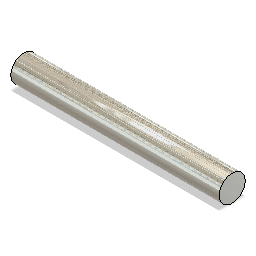
GuardaLamas_1 (Autodesk Fusion 360 archive; units mm, degrees)
design "Shaft2"
Autodesk Fusion 360 part; units mm, degrees
sketch "Sketch1" plane through (0, 0, 0) normal (1, 0, 0) x (0, 0, -1)
  circle A0 centre (0, 0) radius 1.5
  dimension "d1" = 3
  constraint coincident A0.centre origin
  measures "d1" diameter of A0
extrude "Extrude1" add sketch "Sketch1" along normal blind 23.5
extrude "Extrude2" add 1 faces at (0, -0.5383, -0.567) along direction (-1, 0, 0) blind 0.5

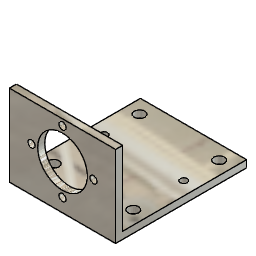
design "chapinhas"
Autodesk Fusion 360 part; units mm, degrees
sketch "Sketch1" plane through (0, 0, 0) normal (0, 0, 1) x (1, 0, 0)
  circle A0 centre (0, 0) radius 14
  circle A1 centre (17.5, 0) radius 2
  circle A2 centre (0, 17.5) radius 2
  circle A3 centre (-17.5, 0) radius 2
  circle A4 centre (0, -17.5) radius 2
  line L0 (30, -21) -> (-30, -21)
  line L1 (-30, -21) -> (-30, 21)
  line L2 (-30, 21) -> (30, 21)
  line L3 (30, 21) -> (30, -21)
  line L4 (-30, -21) -> (30, -21)
  line L5 (30, -21) -> (30, -25)
  line L6 (30, -25) -> (-30, -25)
  line L7 (-30, -25) -> (-30, -21)
  dimension "d2" = 28
  dimension "d4" = 4
  dimension "d6" = 360
  dimension "d7" = 60
  dimension "d8" = 42
  dimension "d9" = 60
  dimension "d10" = 4
  constraint horizontal L0
  constraint perpendicular L0 L1
  constraint parallel L0 L2
  constraint parallel L1 L3
  constraint coincident A0.centre origin
  constraint horizontal L4
  constraint vertical L5
  constraint horizontal L6
  constraint vertical L7
  measures "d2" diameter of A0
  measures "d4" diameter of A1
  measures "d4" distance of L0.end L6.end
extrude "Extrude1" add sketch "Sketch1" along normal blind 4
extrude "Extrude2" add sketch "Sketch1" against normal blind 70 contours L0 L4 L5 L6 L7
sketch "Sketch2" plane through (0, -25, 0) normal (0, -1, 0) x (1, 0, 0)
  line L0 (30, -70) -> (30, 4)
  line L1 (30, 4) -> (-30, 4)
  line L2 (-30, 4) -> (-30, -70)
  line L3 (-30, -70) -> (30, -70)
  circle A0 centre (-22.5, -13.5) radius 3
  circle A1 centre (-22.5, -42) radius 2
  circle A2 centre (-22.5, -62) radius 3
  circle A3 centre (22.5, -42) radius 2
  circle A4 centre (22.5, -62) radius 3
  circle A5 centre (22.5, -13.5) radius 3
  dimension "d24" = 6
  dimension "d25" = 4
  dimension "d26" = 6
  measures "d24" diameter of A0
  measures "d4" diameter of A1
  measures "d26" diameter of A2
extrude "Extrude3" cut sketch "Sketch2" against normal blind 10 contours A0 | A1 | A2 | A3 | A4 | A5
equation "d11 = d10"

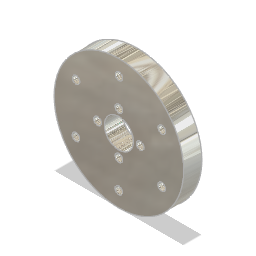
design "Espacador"
Autodesk Fusion 360 part; units mm, degrees
sketch "Sketch1" plane through (0, 0, 0) normal (0, 0, 1) x (-1, 0, 0)
  circle A0 centre (0, 0) radius 9.55
  circle A1 centre (0, 0) radius 32.5
  circle A2 centre (-0.0863, -32.4999) radius 2.5
  circle A3 centre (28.1026, -16.3247) radius 2.5
  circle A4 centre (28.1889, 16.1752) radius 2.5
  circle A5 centre (0.0863, 32.4999) radius 2.5
  circle A6 centre (-28.1026, 16.3247) radius 2.5
  circle A7 centre (-28.1889, -16.1752) radius 2.5
  circle A8 centre (0, 0) radius 42.5
  dimension "d1" = 19.1
  dimension "d4" = 65
  dimension "d5" = 5
  dimension "d7" = 360
  dimension "d9" = 85
  constraint concentric A0 A1
  constraint coincident A1 A2.centre
  constraint concentric A1 A8
  measures "d1" diameter of A0
  measures "d4" diameter of A1
  measures "d5" diameter of A2
  measures "d9" diameter of A8
extrude "Extrude1" add sketch "Sketch1" along normal blind 12 contours A1 A2 A3 A4 A5 A6 A7 | A8
sketch "Sketch2" plane through (0, 0, 12) normal (0, 0, 1) x (1, 0, 0)
  circle A0 centre (28.1026, -16.3247) radius 2.5
  circle A1 centre (0.0863, 32.4999) radius 2.5
  circle A2 centre (-0.0863, -32.4999) radius 2.5
  circle A3 centre (28.1889, 16.1752) radius 2.5
  circle A4 centre (-28.1026, 16.3247) radius 2.5
  circle A5 centre (-28.1889, -16.1752) radius 2.5
  circle A6 centre (0, 0) radius 9.55
  circle A7 centre (0, 0) radius 42.5
  circle A8 centre (0, 0) radius 14
  circle A9 centre (14, 0) radius 2.55
  circle A10 centre (0, 14) radius 2.55
  circle A11 centre (-14, 0) radius 2.55
  circle A12 centre (0, -14) radius 2.55
  dimension "d10" = 28
  dimension "d11" = 5.1
  dimension "d13" = 360
  constraint coincident A6.centre A7.centre
  constraint coincident A8 A9.centre
  measures "d10" diameter of A8
  measures "d11" diameter of A9
extrude "Extrude2" cut sketch "Sketch2" against normal blind 31 contours A8 A9 | A8 A9 | A8 A10 | A8 A10 | A8 A12 | A8 A12 | A8 A11 | A8 A11

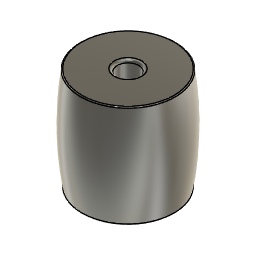
design "Borracha_roda"
Autodesk Fusion 360 part; units mm, degrees
sketch "Esboço1" plane through (0, 0, 0) normal (1, 0, 0) x (0, 1, 0)
  line L0 (0, 0) -> (8.5, 0)
  line L1 (0, 0) -> (0, 19)
  line L2 (0, 19) -> (8.7, 19)
  arc A0 (8.5, 0) -> (8.7, 19) centre (-53.1703, 10.1502) ccw
  line L3 (8.5, 0) -> (8.5, 10.6447)
  dimension "d1" = 8.5
  dimension "d2" = 19
  dimension "d3" = 8.7
  dimension "d5" = 125
  constraint coincident L0.start L1.start
  constraint horizontal L0
  constraint perpendicular L0 L1
  constraint perpendicular L1 L2
  constraint perpendicular L0 L3
  measures "d1" distance of L0.start L0.end
  measures "d2" distance of L0.start L1.end
  measures "d3" distance of L1.end L2.end
  measures "d5" diameter of A0
revolve "Revolucionar1" add sketch "Esboço1" angle 360 about axis through (0, 0, 0) along (0, 0, 1)
sketch "Esboço2" plane through (0, 0, 19) normal (0, 0, 1) x (-1, 0, 0)
  circle A0 centre (0, 0) radius 8.7
  circle A1 centre (0, 0) radius 2
  dimension "d7" = 4
  constraint concentric A0 A1
  measures "d7" diameter of A1
extrude "Extrusão1" cut sketch "Esboço2" against normal blind 24 contours A1
fillet "Arredondamento1" radius 0.5 2 edges at (1.8647, -0.7232, 19) (1.8647, 0.7232, 0)
fillet "Arredondamento2" radius 0.2 2 edges at (-8.1112, 3.1461, 19) (-7.9248, 3.0737, 0)

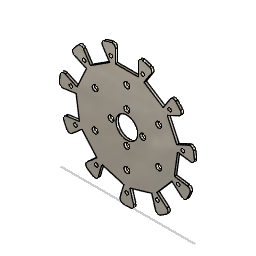
design "Disc Baixo" references "Shaft2"
Autodesk Fusion 360 part; units mm, degrees
sketch "Sketch3" plane through (0, 0, 0) normal (0, 0, 1) x (-1, 0, 0)
  arc A0 (-58.8397, -11.7426) -> (-54.6515, -13.8844) centre (-55.8977, -11.1555) ccw
  line L0 (-54.6515, -13.8844) -> (-44.1121, -9.0712)
  line L1 (-44.1121, -9.0712) -> (-35.7428, -27.3974)
  line L2 (-35.7428, -27.3974) -> (-46.2822, -32.2105)
  arc A1 (-46.2822, -32.2105) -> (-47.4063, -36.7783) centre (-45.036, -34.9394) ccw
  arc A2 (-47.4063, -36.7783) -> (-43.1506, -41.6896) centre (0, 0) ccw
  arc A3 (-43.1506, -41.6896) -> (-38.4693, -41.2271) centre (-40.9931, -39.6052) ccw
  line L3 (-38.4693, -41.2271) -> (-32.2052, -31.48)
  line L4 (-32.2052, -31.48) -> (-15.2567, -42.3722)
  line L5 (-15.2567, -42.3722) -> (-21.5207, -52.1193)
  arc A4 (-21.5207, -52.1193) -> (-19.9968, -56.5697) centre (-18.997, -53.7412) ccw
  arc A5 (-19.9968, -56.5697) -> (-13.7615, -58.4005) centre (0, 0) ccw
  arc A6 (-13.7615, -58.4005) -> (-10.0734, -55.4805) centre (-13.0734, -55.4805) ccw
  line L6 (-10.0734, -55.4805) -> (-10.0734, -43.8941)
  line L7 (-10.0734, -43.8941) -> (10.0734, -43.8941)
  line L8 (10.0734, -43.8941) -> (10.0734, -55.4805)
  arc A7 (10.0734, -55.4805) -> (13.7615, -58.4005) centre (13.0734, -55.4805) ccw
  arc A8 (13.7615, -58.4005) -> (19.9968, -56.5697) centre (0, 0) ccw
  arc A9 (19.9968, -56.5697) -> (21.5207, -52.1193) centre (18.997, -53.7412) ccw
  line L9 (21.5207, -52.1193) -> (15.2567, -42.3722)
  line L10 (15.2567, -42.3722) -> (32.2052, -31.48)
  line L11 (32.2052, -31.48) -> (38.4693, -41.2271)
  arc A10 (38.4693, -41.2271) -> (43.1506, -41.6896) centre (40.9931, -39.6052) ccw
  arc A11 (43.1506, -41.6896) -> (47.4063, -36.7783) centre (0, 0) ccw
  arc A12 (47.4063, -36.7783) -> (46.2822, -32.2105) centre (45.036, -34.9394) ccw
  line L12 (46.2822, -32.2105) -> (35.7428, -27.3974)
  line L13 (35.7428, -27.3974) -> (44.1121, -9.0712)
  line L14 (44.1121, -9.0712) -> (54.6515, -13.8844)
  arc A13 (54.6515, -13.8844) -> (58.8397, -11.7426) centre (55.8977, -11.1555) ccw
  arc A14 (58.8397, -11.7426) -> (59.7646, -5.3101) centre (0, 0) ccw
  arc A15 (59.7646, -5.3101) -> (56.3494, -2.0752) centre (56.7763, -5.0446) ccw
  line L15 (56.3494, -2.0752) -> (44.8809, -3.7241)
  line L16 (44.8809, -3.7241) -> (42.0137, 16.2176)
  line L17 (42.0137, 16.2176) -> (53.4822, 17.8666)
  arc A16 (53.4822, 17.8666) -> (55.8476, 21.9327) centre (53.0553, 20.836) ccw
  arc A17 (55.8476, 21.9327) -> (53.148, 27.844) centre (0, 0) ccw
  arc A18 (53.148, 27.844) -> (48.526, 28.719) centre (50.4906, 26.4518) ccw
  line L18 (48.526, 28.719) -> (39.7696, 21.1316)
  line L19 (39.7696, 21.1316) -> (26.5763, 36.3575)
  line L20 (26.5763, 36.3575) -> (35.3327, 43.945)
  arc A19 (35.3327, 43.945) -> (35.1243, 48.6444) centre (33.3681, 46.2122) ccw
  arc A20 (35.1243, 48.6444) -> (29.6574, 52.1578) centre (0, 0) ccw
  arc A21 (29.6574, 52.1578) -> (25.296, 50.3952) centre (28.1745, 49.55) ccw
  line L21 (25.296, 50.3952) -> (22.0318, 39.2781)
  line L22 (22.0318, 39.2781) -> (2.701, 44.9541)
  line L23 (2.701, 44.9541) -> (5.9653, 56.0712)
  arc A22 (5.9653, 56.0712) -> (3.2493, 59.912) centre (3.0868, 56.9164) ccw
  arc A23 (3.2493, 59.912) -> (-3.2493, 59.912) centre (0, 0) ccw
  arc A24 (-3.2493, 59.912) -> (-5.9653, 56.0712) centre (-3.0868, 56.9164) ccw
  line L24 (-5.9653, 56.0712) -> (-2.701, 44.9541)
  line L25 (-2.701, 44.9541) -> (-22.0318, 39.2781)
  line L26 (-22.0318, 39.2781) -> (-25.296, 50.3952)
  arc A25 (-25.296, 50.3952) -> (-29.6574, 52.1578) centre (-28.1745, 49.55) ccw
  arc A26 (-29.6574, 52.1578) -> (-35.1243, 48.6444) centre (0, 0) ccw
  arc A27 (-35.1243, 48.6444) -> (-35.3327, 43.945) centre (-33.3681, 46.2122) ccw
  line L27 (-35.3327, 43.945) -> (-26.5763, 36.3575)
  line L28 (-26.5763, 36.3575) -> (-39.7696, 21.1316)
  line L29 (-39.7696, 21.1316) -> (-48.526, 28.719)
  arc A28 (-48.526, 28.719) -> (-53.148, 27.844) centre (-50.4906, 26.4518) ccw
  arc A29 (-53.148, 27.844) -> (-55.8476, 21.9327) centre (0, 0) ccw
  arc A30 (-55.8476, 21.9327) -> (-53.4822, 17.8666) centre (-53.0553, 20.836) ccw
  line L30 (-53.4822, 17.8666) -> (-42.0137, 16.2176)
  line L31 (-42.0137, 16.2176) -> (-44.8809, -3.7241)
  line L32 (-44.8809, -3.7241) -> (-56.3494, -2.0752)
  arc A31 (-56.3494, -2.0752) -> (-59.7646, -5.3101) centre (-56.7763, -5.0446) ccw
  arc A32 (-59.7646, -5.3101) -> (-58.8397, -11.7426) centre (0, 0) ccw
  circle A33 centre (-45.4816, 20.7708) radius 1.5
  circle A34 centre (-27.032, 42.0627) radius 1.5
  circle A35 centre (0, 50) radius 1.5
  circle A36 centre (27.032, 42.0627) radius 1.5
  circle A37 centre (45.4816, 20.7708) radius 1.5
  circle A38 centre (49.4911, -7.1157) radius 1.5
  circle A39 centre (37.7875, -32.743) radius 1.5
  circle A40 centre (14.0866, -47.9746) radius 1.5
  circle A41 centre (-49.4911, -7.1157) radius 1.5
  circle A42 centre (-37.7875, -32.743) radius 1.5
  circle A43 centre (-14.0866, -47.9746) radius 1.5
  circle A44 centre (12.5, -21.6506) radius 8
  circle A45 centre (-20.5681, -11.875) radius 2.6
  circle A46 centre (-20.5681, 11.875) radius 2.6
  circle A47 centre (0, 23.75) radius 2.6
  circle A48 centre (20.5681, 11.875) radius 2.6
  circle A49 centre (20.5681, -11.875) radius 2.6
  circle A50 centre (-12.5, -21.6506) radius 8
  circle A51 centre (0, -23.75) radius 2.6
  circle A52 centre (25, 0) radius 8
  circle A53 centre (12.5, 21.6506) radius 8
  circle A54 centre (-12.5, 21.6506) radius 8
  circle A55 centre (-25, 0) radius 8
  circle A56 centre (0, 0) radius 11
  circle A57 centre (0, 50) radius 1.5
extrude "Extrude2" add sketch "Sketch3" along normal blind 2 contours A0 L0 L1 L2 A1 A2 A3 L3 L4 L5 A4 A5 A6 L6 L7 L8 A7 A8 A9 L9 L10 L11 A10 A11 A12 L12 L13 L14 A13 A14 A15 L15 L16 L17 A16 A17 A18 L18 L19 L20 A19 A20 A21 L21 L22 L23 A22 A23 A24 L24 L25 L26 A25 A26 A27 L27 L28 L29 A28 A29 A30 L30 L31 L32 A31 A32 | A33 | A34 | A35 A57 | A36 | A37 | A38 | A39 | A40 | A41 | A42 | A43 | A44 | A45 | A46 | A47 | A48 | A49 | A50 | A51 | A52 | A53 | A54 | A55 | A56
component_pattern "component pattern"
move_body "Move2" bodies 1 to x (1, 0, 0) y (0, 1, 0) z (0, 0, 1) at (0, 0, -2)
combine "Combine3" [suppressed]
sketch "Sketch5" plane through (0, 0, -2) normal (0, 0, -1) x (-1, 0, 0)
  line L0 (54.6515, 13.8844) -> (44.1121, 9.0712)
  line L1 (44.1121, 9.0712) -> (35.7428, 27.3974)
  line L2 (35.7428, 27.3974) -> (46.2822, 32.2105)
  arc A0 (46.2822, 32.2105) -> (47.4063, 36.7783) centre (45.036, 34.9394) ccw
  arc A1 (47.4063, 36.7783) -> (43.1506, 41.6896) centre (0, 0) ccw
  arc A2 (43.1506, 41.6896) -> (38.4693, 41.2271) centre (40.9931, 39.6052) ccw
  line L3 (38.4693, 41.2271) -> (32.2052, 31.48)
  line L4 (32.2052, 31.48) -> (15.2567, 42.3722)
  line L5 (15.2567, 42.3722) -> (21.5207, 52.1193)
  arc A3 (21.5207, 52.1193) -> (19.9968, 56.5697) centre (18.997, 53.7412) ccw
  arc A4 (19.9968, 56.5697) -> (13.7615, 58.4005) centre (0, 0) ccw
  arc A5 (13.7615, 58.4005) -> (10.0734, 55.4805) centre (13.0734, 55.4805) ccw
  line L6 (10.0734, 55.4805) -> (10.0734, 43.8941)
  line L7 (10.0734, 43.8941) -> (-10.0734, 43.8941)
  line L8 (-10.0734, 43.8941) -> (-10.0734, 55.4805)
  arc A6 (-10.0734, 55.4805) -> (-13.7615, 58.4005) centre (-13.0734, 55.4805) ccw
  arc A7 (-13.7615, 58.4005) -> (-19.9968, 56.5697) centre (0, 0) ccw
  arc A8 (-19.9968, 56.5697) -> (-21.5207, 52.1193) centre (-18.997, 53.7412) ccw
  line L9 (-21.5207, 52.1193) -> (-15.2567, 42.3722)
  line L10 (-15.2567, 42.3722) -> (-32.2052, 31.48)
  line L11 (-32.2052, 31.48) -> (-38.4693, 41.2271)
  arc A9 (-38.4693, 41.2271) -> (-43.1506, 41.6896) centre (-40.9931, 39.6052) ccw
  arc A10 (-43.1506, 41.6896) -> (-47.4063, 36.7783) centre (0, 0) ccw
  arc A11 (-47.4063, 36.7783) -> (-46.2822, 32.2105) centre (-45.036, 34.9394) ccw
  line L12 (-46.2822, 32.2105) -> (-35.7428, 27.3974)
  line L13 (-35.7428, 27.3974) -> (-44.1121, 9.0712)
  line L14 (-44.1121, 9.0712) -> (-54.6515, 13.8844)
  arc A12 (-54.6515, 13.8844) -> (-58.8397, 11.7426) centre (-55.8977, 11.1555) ccw
  arc A13 (-58.8397, 11.7426) -> (-59.7646, 5.3101) centre (0, 0) ccw
  arc A14 (-59.7646, 5.3101) -> (-56.3494, 2.0752) centre (-56.7763, 5.0446) ccw
  line L15 (-56.3494, 2.0752) -> (-44.8809, 3.7241)
  line L16 (-44.8809, 3.7241) -> (-42.0137, -16.2176)
  line L17 (-42.0137, -16.2176) -> (-53.4822, -17.8666)
  arc A15 (-53.4822, -17.8666) -> (-55.8476, -21.9327) centre (-53.0553, -20.836) ccw
  arc A16 (-55.8476, -21.9327) -> (-53.148, -27.844) centre (0, 0) ccw
  arc A17 (-53.148, -27.844) -> (-48.526, -28.719) centre (-50.4906, -26.4518) ccw
  line L18 (-48.526, -28.719) -> (-39.7696, -21.1316)
  line L19 (-39.7696, -21.1316) -> (-26.5763, -36.3575)
  line L20 (-26.5763, -36.3575) -> (-35.3327, -43.945)
  arc A18 (-35.3327, -43.945) -> (-35.1243, -48.6444) centre (-33.3681, -46.2122) ccw
  arc A19 (-35.1243, -48.6444) -> (-29.6574, -52.1578) centre (0, 0) ccw
  arc A20 (-29.6574, -52.1578) -> (-25.296, -50.3952) centre (-28.1745, -49.55) ccw
  line L21 (-25.296, -50.3952) -> (-22.0318, -39.2781)
  line L22 (-22.0318, -39.2781) -> (-2.701, -44.9541)
  line L23 (-2.701, -44.9541) -> (-5.9653, -56.0712)
  arc A21 (-5.9653, -56.0712) -> (-3.2493, -59.912) centre (-3.0868, -56.9164) ccw
  arc A22 (-3.2493, -59.912) -> (3.2493, -59.912) centre (0, 0) ccw
  arc A23 (3.2493, -59.912) -> (5.9653, -56.0712) centre (3.0868, -56.9164) ccw
  line L24 (5.9653, -56.0712) -> (2.701, -44.9541)
  line L25 (2.701, -44.9541) -> (22.0318, -39.2781)
  line L26 (22.0318, -39.2781) -> (25.296, -50.3952)
  arc A24 (25.296, -50.3952) -> (29.6574, -52.1578) centre (28.1745, -49.55) ccw
  arc A25 (29.6574, -52.1578) -> (35.1243, -48.6444) centre (0, 0) ccw
  arc A26 (35.1243, -48.6444) -> (35.3327, -43.945) centre (33.3681, -46.2122) ccw
  line L27 (35.3327, -43.945) -> (26.5763, -36.3575)
  line L28 (26.5763, -36.3575) -> (39.7696, -21.1316)
  line L29 (39.7696, -21.1316) -> (48.526, -28.719)
  arc A27 (48.526, -28.719) -> (53.148, -27.844) centre (50.4906, -26.4518) ccw
  arc A28 (53.148, -27.844) -> (55.8476, -21.9327) centre (0, 0) ccw
  arc A29 (55.8476, -21.9327) -> (53.4822, -17.8666) centre (53.0553, -20.836) ccw
  line L30 (53.4822, -17.8666) -> (42.0137, -16.2176)
  line L31 (42.0137, -16.2176) -> (44.8809, 3.7241)
  line L32 (44.8809, 3.7241) -> (56.3494, 2.0752)
  arc A30 (56.3494, 2.0752) -> (59.7646, 5.3101) centre (56.7763, 5.0446) ccw
  arc A31 (59.7646, 5.3101) -> (58.8397, 11.7426) centre (0, 0) ccw
  arc A32 (58.8397, 11.7426) -> (54.6515, 13.8844) centre (55.8977, 11.1555) ccw
  circle A33 centre (0, 0) radius 9.6
  circle A34 centre (0, 0) radius 32.5
  circle A35 centre (0, -32.5) radius 2.55
  circle A36 centre (28.1458, -16.25) radius 2.55
  circle A37 centre (28.1458, 16.25) radius 2.55
  circle A38 centre (0, 32.5) radius 2.55
  circle A39 centre (-28.1458, 16.25) radius 2.55
  circle A40 centre (-28.1458, -16.25) radius 2.55
  dimension "d11" = 19.2
  dimension "d16" = 65
  dimension "d17" = 5.1
  dimension "d19" = 360
  constraint coincident A1.centre A4.centre
  constraint concentric A33 A34
  constraint coincident A34 A35.centre
  measures "d11" diameter of A33
  measures "d16" diameter of A34
  measures "d17" diameter of A35
extrude "Extrude4" cut sketch "Sketch5" against normal blind 10 contours A33 | A34 A37 | A34 A37 | A34 A36 | A34 A36 | A34 A38 | A34 A38 | A34 A35 | A34 A35 | A34 A39 | A34 A39 | A34 A40 | A34 A40
sketch "Sketch6" plane through (0, 0, -2) normal (0, 0, -1) x (-1, 0, 0)
  circle A0 centre (0, 32.5) radius 2.55
  circle A1 centre (0, 0) radius 9.6
  circle A2 centre (28.1458, 16.25) radius 2.55
  circle A3 centre (-28.1458, 16.25) radius 2.55
  circle A4 centre (0, -32.5) radius 2.55
  circle A5 centre (28.1458, -16.25) radius 2.55
  circle A6 centre (-28.1458, -16.25) radius 2.55
  arc A7 (-58.8397, 11.7426) -> (-59.7646, 5.3101) centre (0, 0) ccw
  arc A8 (-59.7646, 5.3101) -> (-56.3494, 2.0752) centre (-56.7763, 5.0446) ccw
  line L0 (-56.3494, 2.0752) -> (-44.8809, 3.7241)
  line L1 (-44.8809, 3.7241) -> (-42.0137, -16.2176)
  line L2 (-42.0137, -16.2176) -> (-53.4822, -17.8666)
  arc A9 (-53.4822, -17.8666) -> (-55.8476, -21.9327) centre (-53.0553, -20.836) ccw
  arc A10 (-55.8476, -21.9327) -> (-53.148, -27.844) centre (0, 0) ccw
  arc A11 (-53.148, -27.844) -> (-48.526, -28.719) centre (-50.4906, -26.4518) ccw
  line L3 (-48.526, -28.719) -> (-39.7696, -21.1316)
  line L4 (-39.7696, -21.1316) -> (-26.5763, -36.3575)
  line L5 (-26.5763, -36.3575) -> (-35.3327, -43.945)
  arc A12 (-35.3327, -43.945) -> (-35.1243, -48.6444) centre (-33.3681, -46.2122) ccw
  arc A13 (-35.1243, -48.6444) -> (-29.6574, -52.1578) centre (0, 0) ccw
  arc A14 (-29.6574, -52.1578) -> (-25.296, -50.3952) centre (-28.1745, -49.55) ccw
  line L6 (-25.296, -50.3952) -> (-22.0318, -39.2781)
  line L7 (-22.0318, -39.2781) -> (-2.701, -44.9541)
  line L8 (-2.701, -44.9541) -> (-5.9653, -56.0712)
  arc A15 (-5.9653, -56.0712) -> (-3.2493, -59.912) centre (-3.0868, -56.9164) ccw
  arc A16 (-3.2493, -59.912) -> (3.2493, -59.912) centre (0, 0) ccw
  arc A17 (3.2493, -59.912) -> (5.9653, -56.0712) centre (3.0868, -56.9164) ccw
  line L9 (5.9653, -56.0712) -> (2.701, -44.9541)
  line L10 (2.701, -44.9541) -> (22.0318, -39.2781)
  line L11 (22.0318, -39.2781) -> (25.296, -50.3952)
  arc A18 (25.296, -50.3952) -> (29.6574, -52.1578) centre (28.1745, -49.55) ccw
  arc A19 (29.6574, -52.1578) -> (35.1243, -48.6444) centre (0, 0) ccw
  arc A20 (35.1243, -48.6444) -> (35.3327, -43.945) centre (33.3681, -46.2122) ccw
  line L12 (35.3327, -43.945) -> (26.5763, -36.3575)
  line L13 (26.5763, -36.3575) -> (39.7696, -21.1316)
  line L14 (39.7696, -21.1316) -> (48.526, -28.719)
  arc A21 (48.526, -28.719) -> (53.148, -27.844) centre (50.4906, -26.4518) ccw
  arc A22 (53.148, -27.844) -> (55.8476, -21.9327) centre (0, 0) ccw
  arc A23 (55.8476, -21.9327) -> (53.4822, -17.8666) centre (53.0553, -20.836) ccw
  line L15 (53.4822, -17.8666) -> (42.0137, -16.2176)
  line L16 (42.0137, -16.2176) -> (44.8809, 3.7241)
  line L17 (44.8809, 3.7241) -> (56.3494, 2.0752)
  arc A24 (56.3494, 2.0752) -> (59.7646, 5.3101) centre (56.7763, 5.0446) ccw
  arc A25 (59.7646, 5.3101) -> (58.8397, 11.7426) centre (0, 0) ccw
  arc A26 (58.8397, 11.7426) -> (54.6515, 13.8844) centre (55.8977, 11.1555) ccw
  line L18 (54.6515, 13.8844) -> (44.1121, 9.0712)
  line L19 (44.1121, 9.0712) -> (35.7428, 27.3974)
  line L20 (35.7428, 27.3974) -> (46.2822, 32.2105)
  arc A27 (46.2822, 32.2105) -> (47.4063, 36.7783) centre (45.036, 34.9394) ccw
  arc A28 (47.4063, 36.7783) -> (43.1506, 41.6896) centre (0, 0) ccw
  arc A29 (43.1506, 41.6896) -> (38.4693, 41.2271) centre (40.9931, 39.6052) ccw
  line L21 (38.4693, 41.2271) -> (32.2052, 31.48)
  line L22 (32.2052, 31.48) -> (15.2567, 42.3722)
  line L23 (15.2567, 42.3722) -> (21.5207, 52.1193)
  arc A30 (21.5207, 52.1193) -> (19.9968, 56.5697) centre (18.997, 53.7412) ccw
  arc A31 (19.9968, 56.5697) -> (13.7615, 58.4005) centre (0, 0) ccw
  arc A32 (13.7615, 58.4005) -> (10.0734, 55.4805) centre (13.0734, 55.4805) ccw
  line L24 (10.0734, 55.4805) -> (10.0734, 43.8941)
  line L25 (10.0734, 43.8941) -> (-10.0734, 43.8941)
  line L26 (-10.0734, 43.8941) -> (-10.0734, 55.4805)
  arc A33 (-10.0734, 55.4805) -> (-13.7615, 58.4005) centre (-13.0734, 55.4805) ccw
  arc A34 (-13.7615, 58.4005) -> (-19.9968, 56.5697) centre (0, 0) ccw
  arc A35 (-19.9968, 56.5697) -> (-21.5207, 52.1193) centre (-18.997, 53.7412) ccw
  line L27 (-21.5207, 52.1193) -> (-15.2567, 42.3722)
  line L28 (-15.2567, 42.3722) -> (-32.2052, 31.48)
  line L29 (-32.2052, 31.48) -> (-38.4693, 41.2271)
  arc A36 (-38.4693, 41.2271) -> (-43.1506, 41.6896) centre (-40.9931, 39.6052) ccw
  arc A37 (-43.1506, 41.6896) -> (-47.4063, 36.7783) centre (0, 0) ccw
  arc A38 (-47.4063, 36.7783) -> (-46.2822, 32.2105) centre (-45.036, 34.9394) ccw
  line L30 (-46.2822, 32.2105) -> (-35.7428, 27.3974)
  line L31 (-35.7428, 27.3974) -> (-44.1121, 9.0712)
  line L32 (-44.1121, 9.0712) -> (-54.6515, 13.8844)
  arc A39 (-54.6515, 13.8844) -> (-58.8397, 11.7426) centre (-55.8977, 11.1555) ccw
  circle A40 centre (0, -50) radius 1.55
  circle A41 centre (27.032, -42.0627) radius 1.55
  circle A42 centre (45.4816, -20.7708) radius 1.55
  circle A43 centre (49.4911, 7.1157) radius 1.55
  circle A44 centre (37.7875, 32.743) radius 1.55
  circle A45 centre (14.0866, 47.9746) radius 1.55
  circle A46 centre (-14.0866, 47.9746) radius 1.55
  circle A47 centre (-37.7875, 32.743) radius 1.55
  circle A48 centre (-49.4911, 7.1157) radius 1.55
  circle A49 centre (-45.4816, -20.7708) radius 1.55
  circle A50 centre (-27.032, -42.0627) radius 1.55
  dimension "d20" = 3.1
  dimension "d22" = 360
  measures "d20" diameter of A40
extrude "Extrude6" cut sketch "Sketch6" against normal blind 20 contours A40 | A41 | A42 | A43 | A44 | A45 | A46 | A47 | A48 | A49 | A50
sketch "Sketch8" plane through (0, 0, 0) normal (0, 0, 1) x (1, 0, 0)
  circle A0 centre (49.4911, 7.1157) radius 1.55
  circle A1 centre (-37.7875, 32.743) radius 1.55
  circle A2 centre (0, -50) radius 1.55
  circle A3 centre (-49.4911, 7.1157) radius 1.55
  circle A4 centre (37.7875, 32.743) radius 1.55
  circle A5 centre (45.4816, -20.7708) radius 1.55
  circle A6 centre (-14.0866, 47.9746) radius 1.55
  circle A7 centre (-27.032, -42.0627) radius 1.55
  circle A8 centre (-45.4816, -20.7708) radius 1.55
  circle A9 centre (14.0866, 47.9746) radius 1.55
  circle A10 centre (27.032, -42.0627) radius 1.55
  circle A11 centre (0, 32.5) radius 2.55
  circle A12 centre (0, 0) radius 9.6
  circle A13 centre (-28.1458, 16.25) radius 2.55
  circle A14 centre (28.1458, 16.25) radius 2.55
  circle A15 centre (0, -32.5) radius 2.55
  circle A16 centre (-28.1458, -16.25) radius 2.55
  circle A17 centre (28.1458, -16.25) radius 2.55
  arc A18 (59.7646, 5.3101) -> (58.8397, 11.7426) centre (0, 0) ccw
  arc A19 (58.8397, 11.7426) -> (54.6515, 13.8844) centre (55.8977, 11.1555) ccw
  line L0 (54.6515, 13.8844) -> (44.1121, 9.0712)
  line L1 (44.1121, 9.0712) -> (35.7428, 27.3974)
  line L2 (35.7428, 27.3974) -> (46.2822, 32.2105)
  arc A20 (46.2822, 32.2105) -> (47.4063, 36.7783) centre (45.036, 34.9394) ccw
  arc A21 (47.4063, 36.7783) -> (43.1506, 41.6896) centre (0, 0) ccw
  arc A22 (43.1506, 41.6896) -> (38.4693, 41.2271) centre (40.9931, 39.6052) ccw
  line L3 (38.4693, 41.2271) -> (32.2052, 31.48)
  line L4 (32.2052, 31.48) -> (15.2567, 42.3722)
  line L5 (15.2567, 42.3722) -> (21.5207, 52.1193)
  arc A23 (21.5207, 52.1193) -> (19.9968, 56.5697) centre (18.997, 53.7412) ccw
  arc A24 (19.9968, 56.5697) -> (13.7615, 58.4005) centre (0, 0) ccw
  arc A25 (13.7615, 58.4005) -> (10.0734, 55.4805) centre (13.0734, 55.4805) ccw
  line L6 (10.0734, 55.4805) -> (10.0734, 43.8941)
  line L7 (10.0734, 43.8941) -> (-10.0734, 43.8941)
  line L8 (-10.0734, 43.8941) -> (-10.0734, 55.4805)
  arc A26 (-10.0734, 55.4805) -> (-13.7615, 58.4005) centre (-13.0734, 55.4805) ccw
  arc A27 (-13.7615, 58.4005) -> (-19.9968, 56.5697) centre (0, 0) ccw
  arc A28 (-19.9968, 56.5697) -> (-21.5207, 52.1193) centre (-18.997, 53.7412) ccw
  line L9 (-21.5207, 52.1193) -> (-15.2567, 42.3722)
  line L10 (-15.2567, 42.3722) -> (-32.2052, 31.48)
  line L11 (-32.2052, 31.48) -> (-38.4693, 41.2271)
  arc A29 (-38.4693, 41.2271) -> (-43.1506, 41.6896) centre (-40.9931, 39.6052) ccw
  arc A30 (-43.1506, 41.6896) -> (-47.4063, 36.7783) centre (0, 0) ccw
  arc A31 (-47.4063, 36.7783) -> (-46.2822, 32.2105) centre (-45.036, 34.9394) ccw
  line L12 (-46.2822, 32.2105) -> (-35.7428, 27.3974)
  line L13 (-35.7428, 27.3974) -> (-44.1121, 9.0712)
  line L14 (-44.1121, 9.0712) -> (-54.6515, 13.8844)
  arc A32 (-54.6515, 13.8844) -> (-58.8397, 11.7426) centre (-55.8977, 11.1555) ccw
  arc A33 (-58.8397, 11.7426) -> (-59.7646, 5.3101) centre (0, 0) ccw
  arc A34 (-59.7646, 5.3101) -> (-56.3494, 2.0752) centre (-56.7763, 5.0446) ccw
  line L15 (-56.3494, 2.0752) -> (-44.8809, 3.7241)
  line L16 (-44.8809, 3.7241) -> (-42.0137, -16.2176)
  line L17 (-42.0137, -16.2176) -> (-53.4822, -17.8666)
  arc A35 (-53.4822, -17.8666) -> (-55.8476, -21.9327) centre (-53.0553, -20.836) ccw
  arc A36 (-55.8476, -21.9327) -> (-53.148, -27.844) centre (0, 0) ccw
  arc A37 (-53.148, -27.844) -> (-48.526, -28.719) centre (-50.4906, -26.4518) ccw
  line L18 (-48.526, -28.719) -> (-39.7696, -21.1316)
  line L19 (-39.7696, -21.1316) -> (-26.5763, -36.3575)
  line L20 (-26.5763, -36.3575) -> (-35.3327, -43.945)
  arc A38 (-35.3327, -43.945) -> (-35.1243, -48.6444) centre (-33.3681, -46.2122) ccw
  arc A39 (-35.1243, -48.6444) -> (-29.6574, -52.1578) centre (0, 0) ccw
  arc A40 (-29.6574, -52.1578) -> (-25.296, -50.3952) centre (-28.1745, -49.55) ccw
  line L21 (-25.296, -50.3952) -> (-22.0318, -39.2781)
  line L22 (-22.0318, -39.2781) -> (-2.701, -44.9541)
  line L23 (-2.701, -44.9541) -> (-5.9653, -56.0712)
  arc A41 (-5.9653, -56.0712) -> (-3.2493, -59.912) centre (-3.0868, -56.9164) ccw
  arc A42 (-3.2493, -59.912) -> (3.2493, -59.912) centre (0, 0) ccw
  arc A43 (3.2493, -59.912) -> (5.9653, -56.0712) centre (3.0868, -56.9164) ccw
  line L24 (5.9653, -56.0712) -> (2.701, -44.9541)
  line L25 (2.701, -44.9541) -> (22.0318, -39.2781)
  line L26 (22.0318, -39.2781) -> (25.296, -50.3952)
  arc A44 (25.296, -50.3952) -> (29.6574, -52.1578) centre (28.1745, -49.55) ccw
  arc A45 (29.6574, -52.1578) -> (35.1243, -48.6444) centre (0, 0) ccw
  arc A46 (35.1243, -48.6444) -> (35.3327, -43.945) centre (33.3681, -46.2122) ccw
  line L27 (35.3327, -43.945) -> (26.5763, -36.3575)
  line L28 (26.5763, -36.3575) -> (39.7696, -21.1316)
  line L29 (39.7696, -21.1316) -> (48.526, -28.719)
  arc A47 (48.526, -28.719) -> (53.148, -27.844) centre (50.4906, -26.4518) ccw
  arc A48 (53.148, -27.844) -> (55.8476, -21.9327) centre (0, 0) ccw
  arc A49 (55.8476, -21.9327) -> (53.4822, -17.8666) centre (53.0553, -20.836) ccw
  line L30 (53.4822, -17.8666) -> (42.0137, -16.2176)
  line L31 (42.0137, -16.2176) -> (44.8809, 3.7241)
  line L32 (44.8809, 3.7241) -> (56.3494, 2.0752)
  arc A50 (56.3494, 2.0752) -> (59.7646, 5.3101) centre (56.7763, 5.0446) ccw
  circle A51 centre (0, 0) radius 14
  circle A52 centre (14, 0) radius 2.55
  circle A53 centre (0, 14) radius 2.55
  circle A54 centre (-14, 0) radius 2.55
  circle A55 centre (0, -14) radius 2.55
  dimension "d25" = 28
  dimension "d26" = 5.1
  dimension "d28" = 360
  constraint coincident A12.centre A18.centre
  constraint coincident A51 A52.centre
  measures "d25" diameter of A51
  measures "d26" diameter of A52
extrude "Extrude7" cut sketch "Sketch8" against normal blind 16 contours A51 A52 | A51 A52 | A51 A53 | A51 A53 | A51 A55 | A51 A55 | A51 A54 | A51 A54
